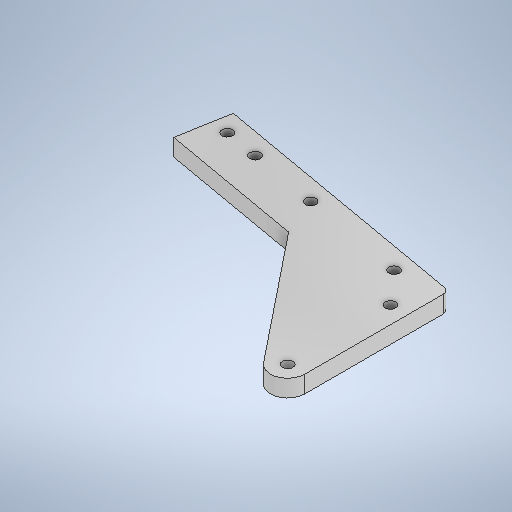
# Autodesk Inventor part: hand2_10
Saved by Autodesk Inventor 2025.1 (Build 291241000, 241)
## iProperties
Created: 2025-02-03
Part Number: hand2_10
Material: アルミニウム 6061-AHC
Document SubType Name: Modeling
Designer: ryogo
Density: 2.7 g/cm^3
Appearance: アルミニウム - ダーク
Author: ryogo
Autodesk Inventor part; units mm, degrees
ref_plane "YZ Plane" through (0, 0, 0) normal (1, 0, 0) x (0, 1, 0)
ref_plane "XZ Plane" through (0, 0, 0) normal (0, 1, 0) x (-1, 0, 0)
ref_plane "XY Plane" through (0, 0, 0) normal (0, 0, 1) x (1, 0, 0)
sketch "スケッチ1" plane through (0, 0, 0) normal (0, 1, 0) x (-1, 0, 0)
  circle A0 centre (0, 0) radius 122.5
  line L0 (0, 0) -> (21.2719, 120.6389)
  line L1 (21.2719, 120.6389) -> (-21.2719, -120.6389)
  line L2 (21.2719, 120.6389) -> (-41.166, -233.4643)
  arc A1 (21.2719, 120.6389) -> (0, 122.5) centre (0, 0) ccw
  arc A2 (-21.2719, -120.6389) -> (0, -122.5) centre (0, 0) ccw
  arc A3 (-41.8975, -115.1123) -> (-21.2719, -120.6389) centre (0, 0) ccw
  circle A4 centre (0, 0) radius 125
  circle A5 centre (0, 0) radius 145
  arc A6 (-42.7525, -117.4616) -> (-105.9051, -66.4011) centre (0, 0) ccw
  line L3 (0, 0) -> (-42.7525, -117.4616) construction
  line L4 (21.706, 123.101) -> (21.706, 123.101)
  line L5 (0, -145) -> (0, -265.735)
  line L6 (0, 0) -> (-41.8975, -115.1123)
  line L7 (-49.5929, -136.2554) -> (-41.8975, -115.1123)
  line L8 (-42.7525, -117.4616) -> (-231.4975, -48.764)
  line L9 (42.7525, 117.4616) -> (0, 0)
  line L10 (0, -145) -> (0, 145)
  line L11 (0, 0) -> (0, 300)
  circle A7 centre (0, 300) radius 20
  line L12 (117.0937, 43.75) -> (18.735, 307)
  line L13 (0, 0) -> (185.4327, 0)
  line L14 (0, 0) -> (-259.4726, 94.4403)
  line L15 (42.7525, 117.4616) -> (-253.7236, 225.3701)
  line L16 (0, 125) -> (22.0409, 125)
  line L17 (21.2719, 120.6389) -> (25.179, 142.7971)
  line L18 (42.7525, 117.4616) -> (65.8461, 180.9106)
  line L19 (15, 170) -> (69.9226, 170)
  line L20 (15.9946, 175) -> (68.0545, 175)
  line L21 (0, 125) -> (-15, 125)
  line L22 (-15, 125) -> (-15, 325)
  line L23 (-15, 325) -> (0, 325)
  line L24 (0, 325) -> (0, 125)
  line L25 (0, 125) -> (15, 125)
  line L26 (15, 125) -> (15, 325)
  line L27 (15, 325) -> (0, 325)
  line L28 (0, 325) -> (0, 125)
  line L29 (15, 200) -> (15, 325)
  line L30 (15, 325) -> (-15, 325)
  line L31 (-15, 325) -> (-15, 150)
  line L32 (15, 170) -> (37.5, 170)
  line L33 (37.5, 170) -> (17.5, 170)
  line L34 (0, 0) -> (0, 300)
  line L35 (0, -125) -> (42.7525, 117.4616)
  line L36 (-42.7525, -117.4616) -> (0, 125)
  line L37 (0, -125) -> (-3.519, -144.9573)
  line L38 (42.7525, 117.4616) -> (49.5929, 136.2554)
  line L39 (0, 125) -> (3.519, 144.9573)
  line L40 (-42.7525, -117.4616) -> (-46.2715, -137.4189)
  line L41 (42.7525, 117.4616) -> (46.2715, 137.4189)
  line L42 (-3.519, -144.9573) -> (46.2715, 137.4189)
  line L43 (46.2715, 137.4189) -> (37.2054, 139.0175)
  line L44 (-12.5852, -143.3587) -> (-3.519, -144.9573)
  line L45 (-46.2715, -137.4189) -> (3.519, 144.9573)
  line L46 (3.519, 144.9573) -> (12.5852, 143.3587)
  line L47 (-37.2054, -139.0175) -> (-46.2715, -137.4189)
  line L48 (-27.6373, -142.3418) -> (-22.7132, -143.21)
  line L49 (-27.6373, -142.3418) -> (-22.7132, -143.21)
  line L50 (-22.7132, -143.21) -> (27.641, 142.363)
  line L51 (27.641, 142.363) -> (22.717, 143.2312)
  line L52 (22.717, 143.2312) -> (-27.6373, -142.3418)
  line L53 (12.5852, 143.3587) -> (-37.2054, -139.0175)
  line L54 (-12.5852, -143.3587) -> (37.2054, 139.0175)
  line L55 (-42.1294, -138.1492) -> (7.6611, 144.2269)
  line L56 (-7.6611, -144.2269) -> (42.1294, 138.1492)
  line L57 (12.5852, 143.3587) -> (7.6611, 144.2269)
  line L58 (7.6611, 144.2269) -> (29.236, 266.5842)
  line L59 (29.236, 266.5842) -> (34.1601, 265.7159)
  line L60 (34.1601, 265.7159) -> (12.5852, 143.3587)
  line L61 (22.717, 143.2312) -> (25.179, 142.7971)
  line L62 (25.179, 142.7971) -> (42.462, 240.8141)
  line L63 (42.462, 240.8141) -> (40, 241.2482)
  line L64 (40, 241.2482) -> (22.717, 143.2312)
  line L65 (42.1294, 138.1492) -> (37.2054, 139.0175)
  line L66 (37.2054, 139.0175) -> (49.9319, 211.1932)
  line L67 (49.9319, 211.1932) -> (54.8559, 210.3249)
  line L68 (54.8559, 210.3249) -> (42.1294, 138.1492)
  line L69 (25.179, 142.7971) -> (27.641, 142.363)
  line L70 (27.641, 142.363) -> (44.508, 238.0204)
  line L71 (44.508, 238.0204) -> (42.046, 238.4546)
  line L72 (42.046, 238.4546) -> (25.179, 142.7971)
  line L73 (15.9946, 175) -> (15, 175)
  line L74 (15, 175) -> (0, 175)
  line L75 (0, 175) -> (0, 170)
  line L76 (0, 170) -> (15, 170)
  line L77 (15, 170) -> (15, 175)
  line L78 (20, 175) -> (40, 175)
  line L79 (40, 175) -> (40, 245)
  line L80 (40, 245) -> (20, 245)
  line L81 (20, 245) -> (20, 175)
  line L82 (0, 175) -> (58.7137, 175)
  line L83 (58.7137, 175) -> (58.7137, 200)
  line L84 (58.7137, 200) -> (0, 200)
  line L85 (0, 200) -> (0, 175)
  line L86 (0, 200) -> (50, 200)
  line L87 (50, 200) -> (50, 170)
  line L88 (50, 170) -> (0, 170)
  line L89 (0, 170) -> (0, 200)
  line L90 (50, 170) -> (0, 170)
  line L91 (0, 170) -> (0, 165)
  line L92 (0, 200) -> (-15, 200)
  line L93 (-15, 200) -> (-15, 180)
  line L94 (-15, 180) -> (0, 180)
  line L95 (0, 180) -> (0, 200)
  line L96 (0, 180) -> (-15, 180)
  line L97 (-15, 180) -> (-15, 175)
  line L98 (-15, 175) -> (0, 175)
  line L99 (0, 175) -> (0, 180)
  line L100 (0, 145) -> (-15, 145)
  line L101 (-15, 145) -> (-20.5, 145)
  line L102 (-20.5, 145) -> (-20.5, 200)
  line L103 (-20.5, 200) -> (-15, 200)
  line L104 (-15, 200) -> (-15, 145)
  line L105 (-20.5, 150) -> (-25, 150)
  line L106 (-25, 150) -> (-25, 180)
  line L107 (-25, 180) -> (-20.5, 180)
  line L108 (-20.5, 180) -> (-20.5, 150)
  line L109 (50, 175) -> (-15, 175)
  line L110 (-15, 175) -> (-15, 170)
  line L111 (50, 170) -> (50, 175)
  line L112 (-20.5, 170) -> (-25, 170)
  line L113 (-25, 170) -> (-25, 200)
  line L114 (-25, 200) -> (-20.5, 200)
  line L115 (-20.5, 200) -> (-20.5, 170)
  line L116 (15, 250) -> (-15, 250)
  line L117 (-15, 145) -> (15, 145)
  line L118 (31.698, 266.1501) -> (-39.6674, -138.5834)
  line L119 (52.3939, 210.7591) -> (-10.1232, -143.7928)
  line L120 (49.3441, 179.0659) -> (14.8758, 185.1436)
  line L121 (-15, 138.4818) -> (-15, 121.5782)
  line L122 (-7.6611, -144.2269) -> (-42.1294, -138.1492)
  line L123 (-39.6243, -123.9424) -> (-5.1561, -130.02)
  line L124 (-42.2291, -138.7145) -> (-7.7608, -144.7922)
  line L125 (-41.3608, -133.7904) -> (-6.8926, -139.8681)
  line L126 (-6.0243, -134.9441) -> (-40.4926, -128.8664)
  line L127 (18.3488, 204.8397) -> (52.8171, 198.762)
  line L128 (50.2124, 183.9899) -> (45.0029, 154.4457)
  line L129 (10.5346, 160.5234) -> (15.7441, 190.0676)
  line L130 (19.217, 209.7638) -> (53.6853, 203.6861)
  line L131 (15, 250) -> (53.6853, 203.6861)
  line L132 (53.6853, 203.6861) -> (53.6853, 170)
  line L133 (53.6853, 170) -> (-15, 170)
  line L134 (-15, 172.5) -> (53.6853, 172.5)
  line L135 (15, 170) -> (15, 150)
  line L136 (15, 150) -> (-15, 150)
  line L137 (-15, 170) -> (15, 170)
  line L138 (15, 150) -> (-15, 150)
  line L139 (-15, 150) -> (-15, 325)
  line L140 (-15, 325) -> (15, 325)
  line L141 (15, 325) -> (15, 150)
  circle A8 centre (0, 300) radius 6
  circle A9 centre (0, 300) radius 11
  line L142 (47.7456, 170) -> (15, 150)
  line L143 (-25, 170) -> (-30, 170)
  line L144 (-30, 170) -> (-30, 140)
  line L145 (-30, 140) -> (-25, 140)
  line L146 (-25, 140) -> (-25, 170)
  line L147 (30, 175) -> (30, 118.7697)
  line L148 (30, 147) -> (30, 132)
  line L149 (-30, 170) -> (-25, 170)
  line L150 (-25, 170) -> (-25, 180)
  line L151 (-25, 180) -> (-30, 180)
  line L152 (-30, 180) -> (-30, 170)
  circle A10 centre (30, 127) radius 1.55
  line L153 (-27.5, 140) -> (-27.5, 180)
  circle A11 centre (-27.5, 145) radius 1.55
  circle A12 centre (-27.5, 175) radius 1.55
  circle A13 centre (-27.5, 145) radius 5
  circle A14 centre (-27.5, 175) radius 5
  circle A15 centre (30, 127) radius 5
  line L154 (28.5063, 122.2283) -> (-28.9937, 140.2283)
  line L155 (-32.5, 145) -> (-32.5, 175)
  line L156 (-24.2958, 178.8384) -> (33.2042, 130.8384)
  line L157 (0, -125) -> (227.9227, -125)
  line L158 (0, 125) -> (227.9227, 125)
  point P0 (-25.1752, -142.7759)
  point P1 (42.3116, 114.9608)
  point P2 (0, 133.0222)
  point P3 (-38.8988, -134.2246)
  point P4 (-38.0306, -129.3005)
  point P5 (-23.2585, -131.9052)
  point P6 (-24.1267, -136.8293)
  point P7 (-9.3546, -139.434)
  point P8 (-8.4863, -134.51)
  point P9 (17.3379, 184.7094)
  point P10 (32.11, 182.1047)
  point P11 (46.8821, 179.5)
  point P12 (50.3551, 199.1962)
  point P13 (35.5829, 201.8009)
  point P14 (20.8108, 204.4056)
  point P15 (0, 240)
  point P16 (0, 190)
  point P17 (0, 289)
  point P18 (0, 311)
  point P19 (37.5, 172.5)
  point P20 (22.5, 172.5)
  point P21 (0, 125)
  point P22 (0, 122.5)
  point P23 (38.2879, 116.3628)
  point P24 (38.7264, 118.8498)
  point P25 (42.3116, 114.9608)
  point P26 (30, 122)
  point P27 (30, 137)
  point P28 (30, 122)
  point P29 (17.511, 143.9387)
  point P30 (15, 144.2221)
  point P31 (15, 146.0349)
  dimension "d0" = 245
  dimension "d7" = 290
  dimension "d19" = 40
  dimension "d1" = 0
  dimension "d4" = 42.5438
  dimension "d5" = 21.3532
  dimension "d6" = 250
  dimension "d10" = 0
  dimension "d12" = 0
  dimension "d13" = 10
  dimension "d15" = 0
  dimension "d16" = 9.8877
  dimension "d18" = 10
  dimension "d21" = 145
  dimension "d23" = 175
  dimension "d26" = 7.5384
  dimension "d30" = 180
  dimension "d34" = 180
  dimension "d35" = 45
  dimension "d37" = 5
  dimension "d38" = 15
  dimension "d39" = 200
  dimension "d40" = 15
  dimension "d41" = 200
  dimension "d47" = 300
  dimension "d52" = 5
  dimension "d53" = 0
  dimension "d54" = 10
  dimension "d55" = 10
  dimension "d56" = 5
  dimension "d57" = 5
  dimension "d60" = 5
  dimension "d61" = 20
  dimension "d62" = 70
  dimension "d63" = 5
  dimension "d65" = 25
  dimension "d66" = 50
  dimension "d68" = 20
  dimension "d69" = 5
  dimension "d74" = 20
  dimension "d75" = 5.5
  dimension "d76" = 55
  dimension "d77" = 4.5
  dimension "d78" = 30
  dimension "d79" = 5
  dimension "d82" = 20
  dimension "d83" = 50
  dimension "d87" = 16.9036
  dimension "d88" = 10.0392
  dimension "d89" = 10.5222
  dimension "d92" = 15
  dimension "d93" = 5
  dimension "d94" = 5
  dimension "d96" = 4.5
  dimension "d97" = 5
  dimension "d98" = 30
  dimension "d99" = 10
  dimension "d101" = 20
  dimension "d102" = 10
  dimension "d103" = 20
  dimension "d104" = 12
  dimension "d105" = 22
  dimension "d106" = 7.5
  dimension "d107" = 15
  dimension "d108" = 30
  dimension "d112" = 5
  dimension "d122" = 10
  constraints: 317 end point, 97 point on line, 48 parallel, 43 perpendicular, 22 horizontal, 22 point on circle, 15 coincident, 14 midpoint, 13 centre point, 9 collinear, 8 tangent, 2 vertical, 1 symmetric about line, 43 other
  measures "d1" horizontal distance of point (0, 0) A2.end
  measures "d4" distance of L6.end A2.end
  measures "d5" distance of A1.end L0.end
  measures "d6" diameter of A4
  measures "d10" horizontal distance of A4.centre L16.start
  measures "d12" distance from line of L5 point (0, 0)
  measures "d15" horizontal distance of A2.end L35.start
  measures "d16" vertical distance of L6.end L35.start
  measures "d18" angle of L9 L1
  measures "d21" distance of L5.start A2.centre
  measures "d23" distance of L11.end L16.start
  measures "d26" distance from line of L15 L16.start
  measures "d30" angle of L4 L17
  measures "d34" angle of L9 L18
  measures "d35" distance from line of L19 L16.start
  measures "d37" distance between parallel lines of L19 L20
  measures "d38" distance of L22.end L23.end
  measures "d39" distance of L21.end L22.end
  measures "d40" distance of L27.end L26.end
  measures "d41" distance from line of L16.start L27
  measures "d47" distance of L3.start L11.end
  measures "d52" distance of L48.start L48.end
  measures "d53" distance from line of L2 point (-25.175, -142.776)
  measures "d54" distance between parallel lines of L52 L53
  measures "d55" distance between parallel lines of L54 L50
  measures "d56" distance of L46.end L55.end
  measures "d57" distance of L43.end L56.end
  measures "d60" distance between parallel lines of L76 L74
  measures "d61" distance of L80.end L79.end
  measures "d62" distance of L79.end L78.end
  measures "d63" distance between parallel lines of L26 L81
  measures "d65" distance of L83.end L82.end
  measures "d66" distance of L87.end L88.end
  measures "d68" distance between parallel lines of L94 L92
  measures "d69" distance between parallel lines of L98 L96
  measures "d74" distance of L16.start L100.start
  measures "d75" distance of L102.end L103.end
  measures "d76" distance of L101.end L102.end
  measures "d77" distance of L106.end L107.end
  measures "d78" distance of L105.end L106.end
  measures "d79" distance between parallel lines of L101 L105
  measures "d82" distance between parallel lines of L105 L112
  measures "d83" distance between parallel lines of L92 L116
  measures "d87" distance of L121.start L121.end
  measures "d88" vertical distance of point (42.312, 114.961) L25.end
  measures "d89" distance of A1.end point (0, 133.022)
  measures "d92" distance of L124.start L123.start
  measures "d93" distance of L124.start L125.start
  measures "d94" distance of L126.end L123.start
  measures "d96" distance from line of L20 point (46.882, 179.5)
  measures "d97" distance of L120.end L129.end
  measures "d98" distance of L128.start L128.end
  measures "d99" distance from line of L116 point (0, 240)
  measures "d101" distance of L127.start L120.end
  measures "d102" diameter of L130 L127
  measures "d103" distance of L19.start L135.end
  measures "d104" diameter of A8
  measures "d105" diameter of A9
  measures "d106" distance from line of point (22.5, 172.5) L141
  measures "d107" distance of point (22.5, 172.5) point (37.5, 172.5)
  measures "d108" distance between parallel lines of L112 L114
  measures "d112" distance of L145.end L144.end
  measures "d122" distance between parallel lines of L145 L105
extrude "押し出し2" add sketch "スケッチ1" against normal blind 5 contours A15 L147 L15 | L15 L147 L158 A15 | A15 L15 L147 | L15 A15 L158 L147 | L158 L147 A10 A15 | L154 L17 L15 L50 | L50 L15 A15 L154 | L15 L50 L158 A15 | L158 A15 L50 L147 A10 | L154 L16 L17 | L15 L158 L50 | L158 L50 A15 | A15 L147 L156 | L147 A15 L50 L156 | L16 L154 L52 L15 | L15 L52 L156 L17 | L17 L156 L50 A15 L158 | A15 L50 | L154 L26 L15 L52 | L15 L26 A5 L156 L52 | L154 L118 L15 L53 | L53 L15 L26 L154 | L15 L53 L60 A5 L26 | A5 L26 L156 | L154 L55 L15 L118 | L15 L118 L46 L53 | A5 L60 L117 L26 | L26 L117 L60 L156 | A13 L15 L144 A5 | A5 L144 A13 | L154 L22 L15 L10 | L10 L15 L39 L154 | L39 L15 L55 L154 | L15 L55 L46 L118 | L46 L118 A5 L60 | A5 L118 L117 L60 | L60 L117 L118 L156 | L144 L15 L153 A5 | A5 L153 A13 L144 | A13 L144 L15 | L15 L22 A5 L10 | L10 A5 L39 L15 | L154 L145 L146 A13 L15 L22 | L39 L46 L55 L15 | L46 L58 A5 L118 | A5 L58 L117 L118 | L118 L117 L58 L136 L156 | L153 L15 A5 | A5 L15 L146 A13 L153 | L144 A13 L153 A11 L15 | L155 A14 L152 L144 A13 | A13 L145 L154 | L117 L58 A5 | L100 L22 L136 L11 | A5 L22 L100 | L11 L136 L58 L117 | L15 A13 A5 L22 | A5 L58 L46 | L136 L58 L156 | L15 L153 A11 A13 L146 A5 | A5 L146 L15 | A13 L146 L145 | L144 L143 L153 A13 | A14 L152 | A5 A13 L146 L105 L102 L101 L22 | L136 L22 L133 L156 L11 | L11 L156 L58 L136 | L101 L102 L156 L22 | A13 L146 L15 | L15 L146 A5 A13 | L146 A13 A5 | L152 A14 L143 | L153 L143 L106 L146 A13 | A14 L153 A12 L152 | A14 L106 L143 | L153 A12 A14 L106 | L133 L22 L156 | L105 L106 L112 L102 | L106 A14 L156 L102 L112 | L106 A14
sketch "スケッチ3" plane through (0, 0, 0) normal (0, 1, 0) x (1, 0, 0)
  arc A0 (24.2958, -178.8384) -> (32.5, -175) centre (27.5, -175) ccw projected
  line L0 (32.5, -175) -> (32.5, -145) projected
  arc A1 (32.5, -145) -> (28.9937, -140.2283) centre (27.5, -145) ccw projected
  line L1 (28.9937, -140.2283) -> (-28.5063, -122.2283) projected
  arc A2 (-28.5063, -122.2283) -> (-33.2042, -130.8384) centre (-30, -127) ccw projected
  line L2 (-33.2042, -130.8384) -> (24.2958, -178.8384) projected
  circle A3 centre (-30, -127) radius 1.55 projected
  circle A4 centre (27.5, -175) radius 1.55 projected
  circle A5 centre (27.5, -145) radius 1.55 projected
  circle A6 centre (-30, -127) radius 5
  circle A7 centre (27.5, -145) radius 5
  line L3 (26.0063, -149.7717) -> (-31.4937, -131.7717)
  circle A8 centre (27.5, -175) radius 5
  line L4 (22.5, -175) -> (22.5, -145)
  line L5 (-7.5, -139.2827) -> (23.5968, -178.1249)
  point P0 (0, 0)
  point P1 (24.2958, -178.8384)
  dimension "d138" = 40
  constraints: 6 end point, 5 point on circle, 5 tangent, 3 coincident, 2 centre point, 1 point on line, 5 other
  measures "d138" distance from line of L0 L5.start
extrude "押し出し3" cut sketch "スケッチ3" against normal blind 5 contours L2 A6 L3 L5 A8
sketch "スケッチ4" plane through (0, 0, 0) normal (0, 1, 0) x (1, 0, 0)
  arc A0 (-28.5063, -122.2283) -> (-31.4937, -131.7717) centre (-30, -127) ccw projected
  line L0 (-29.1318, -122.076) -> (32.5, -132.9433)
  circle A1 centre (-30, -127) radius 1.55 projected
  line L1 (-30, -127) -> (-13.2635, -127)
  line L2 (-28.5063, -122.2283) -> (28.9937, -140.2283) projected
  arc A2 (-28.5063, -122.2283) -> (-31.4937, -131.7717) centre (-30, -127) ccw projected
  arc A3 (32.5, -145) -> (28.9937, -140.2283) centre (27.5, -145) ccw projected
  line L3 (32.5, -145) -> (32.5, -132.9433)
  point P0 (0, 0)
  dimension "d141" = 10
  constraints: 6 end point, 2 tangent, 1 horizontal, 1 point on circle, 1 point on line, 1 vertical
  measures "d141" angle of L0 L1
extrude "押し出し4" add sketch "スケッチ4" against normal blind 5 contours A0 L0 L3 A3 L2
fillet "フィレット1" radius 2 1 edges at (32.5, -2.5, 132.9433)
sketch "スケッチ6" plane through (0, 0, 0) normal (0, 1, 0) x (1, 0, 0)
  circle A0 centre (27.5, -145) radius 1.55 projected
  circle A1 centre (19.2404, -135.6824) radius 1.55
  line L0 (32.5, -175) -> (32.5, -134.6215) projected
  line L1 (30.8473, -132.6519) -> (-29.1318, -122.076) projected
  circle A2 centre (-30, -127) radius 1.55 projected
  point P0 (0, 0)
  dimension "d148" = 3.1
  dimension "d152" = 5
  dimension "d160" = 50
  constraints: 1 centre point, 1 coincident
  measures "d148" diameter of A1
  measures "d152" distance from line of L1 A1.centre
  measures "d160" distance between centres of A2 A1
extrude "押し出し6" cut sketch "スケッチ6" against normal blind 5 contours A1
sketch "スケッチ7" plane through (0, 0, 0) normal (0, 1, 0) x (1, 0, 0)
  arc A0 (-29.1318, -122.076) -> (-31.4937, -131.7717) centre (-30, -127) ccw projected
  circle A1 centre (-30, -127) radius 1.55 projected
  line L0 (-30, -127) -> (-30.554, -130.1418)
  line L1 (30.8473, -132.6519) -> (-29.1318, -122.076) projected
  line L2 (-34.924, -126.1318) -> (-35.7923, -131.0558)
  arc A2 (-35.7923, -131.0558) -> (-31.7365, -136.8481) centre (-30.8682, -131.924) ccw
  line L3 (-31.7365, -136.8481) -> (5.9503, -143.4933)
  line L4 (-7.5, -139.2827) -> (-31.4937, -131.7717) projected
  line L5 (-7.5, -139.2827) -> (23.5968, -178.1249) projected
  point P0 (0, 0)
  point P1 (-5.7858, -141.4239)
  dimension "d155" = 90
  dimension "d156" = 5
  dimension "d157" = 5
  constraints: 6 end point, 3 point on circle, 3 point on line, 2 parallel, 1 centre point, 1 tangent
  measures "d155" angle of L1 L0
  measures "d156" distance of L2.start L2.end
  measures "d157" distance of A0.centre A2.centre
extrude "押し出し7" add sketch "スケッチ7" against normal blind 5 contours A0 L4 L5 L3 A2 L2
sketch "スケッチ8" plane through (0, 0, 0) normal (0, 1, 0) x (1, 0, 0)
  line L0 (-29.1318, -122.076) -> (30.8473, -132.6519) projected
  line L1 (-29.1318, -122.076) -> (-43.9039, -119.4712)
  line L2 (-43.9039, -119.4712) -> (-46.5086, -134.2434)
  line L3 (-5.7858, -141.4239) -> (-31.7365, -136.8481) projected
  line L4 (-31.7365, -136.8481) -> (-46.5086, -134.2434)
  line L5 (-34.924, -126.1318) -> (-35.7923, -131.0558) projected
  circle A0 centre (19.2404, -135.6824) radius 1.55 projected
  arc A1 (32.5, -134.6215) -> (30.8473, -132.6519) centre (30.5, -134.6215) ccw projected
  line L6 (30.8473, -132.6519) -> (-29.1318, -122.076) projected
  arc A2 (-29.1318, -122.076) -> (-34.924, -126.1318) centre (-30, -127) ccw projected
  line L7 (-34.924, -126.1318) -> (-35.7923, -131.0558) projected
  arc A3 (-35.7923, -131.0558) -> (-31.7365, -136.8481) centre (-30.8682, -131.924) ccw projected
  line L8 (-31.7365, -136.8481) -> (-5.7858, -141.4239) projected
  line L9 (-5.7858, -141.4239) -> (23.5968, -178.1249) projected
  arc A4 (23.5968, -178.1249) -> (32.5, -175) centre (27.5, -175) ccw projected
  line L10 (32.5, -175) -> (32.5, -134.6215) projected
  circle A5 centre (-30, -127) radius 1.55 projected
  circle A6 centre (27.5, -175) radius 1.55 projected
  circle A7 centre (27.5, -145) radius 1.55 projected
  point P0 (0, 0)
  dimension "d161" = 10
  constraints: 6 end point, 2 perpendicular, 1 collinear, 1 point on line
  measures "d161" distance between parallel lines of L2 L5
extrude "押し出し8" add sketch "スケッチ8" against normal blind 5 contours A2 L5 A3 L4 L2 L1
sketch "スケッチ9" plane through (0, 0, 0) normal (0, 1, 0) x (1, 0, 0)
  circle A0 centre (19.2404, -135.6824) radius 1.55 projected
  line L0 (19.2404, -135.6824) -> (-44.7721, -124.3953)
  line L1 (-46.5086, -134.2434) -> (-43.9039, -119.4712) projected
  circle A1 centre (-30, -127) radius 1.55 projected
  point P0 (0, 0)
  point P1 (-46.1613, -132.2737)
  point P2 (-44.2512, -121.4409)
  point P3 (-10.3038, -130.473)
  point P4 (-39.8481, -125.2635)
  dimension "d165" = 90
  dimension "d166" = 20
  dimension "d167" = 10
  constraints: 3 point on line, 2 end point
  measures "d165" angle of L1 L0
  measures "d166" distance of point (-10.304, -130.473) A1.centre
  measures "d167" distance of A1.centre point (-39.848, -125.264)
hole "穴1" at (-10.3038, 0, 130.473) at (-39.8481, 0, 125.2635) direction (0, -1, 0) diameter 3.1 end through all
sketch "スケッチ10" plane through (0, 0, 0) normal (0, 1, 0) x (1, 0, 0)
  line L0 (-43.9039, -119.4712) -> (30.8473, -132.6519) projected
  line L1 (-43.9039, -119.4712) -> (-66.5086, -119.4712)
  line L2 (-5.7858, -141.4239) -> (-46.5086, -134.2434) projected
  line L3 (-46.5086, -134.2434) -> (-66.5086, -134.2434)
  line L4 (-66.5086, -119.4712) -> (-66.5086, -134.2434)
  point P0 (0, 0)
  dimension "d175" = 20
  constraints: 6 end point, 2 horizontal, 1 vertical
  measures "d175" distance from line of L2.end L4
equation "\"d18\" = d13"
